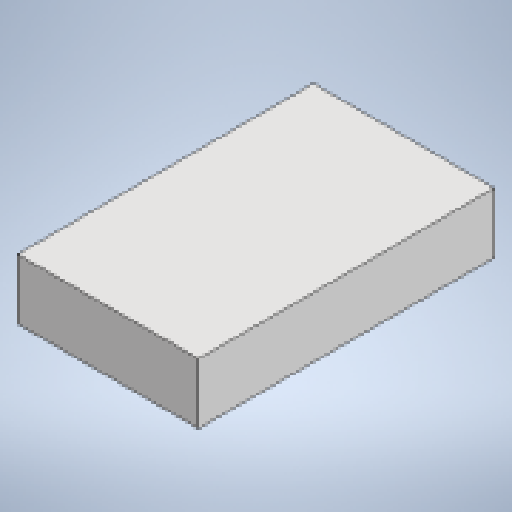
# Autodesk Inventor part: Temp - ESC
Saved by Autodesk Inventor 2023.2 (Build 272271000, 271)
## iProperties
Created: 2023-11-13
Part Number: Temp - ESC
Material: Generic
Document SubType Name: Modeling
Designer: Nathan Cai
Density: 1 g/cm^3
Appearance: Default
Author: Nathan Cai
Autodesk Inventor part; units mm, degrees
ref_plane "YZ Plane" through (0, 0, 0) normal (1, 0, 0) x (0, 1, 0)
ref_plane "XZ Plane" through (0, 0, 0) normal (0, 1, 0) x (-1, 0, 0)
ref_plane "XY Plane" through (0, 0, 0) normal (0, 0, 1) x (1, 0, 0)
sketch "Sketch1" plane through (0, 0, 0) normal (0, 1, 0) x (-1, 0, 0)
  line L0 (-15, 24.5) -> (15, 24.5)
  line L1 (15, 24.5) -> (15, -24.5)
  line L2 (15, -24.5) -> (-15, -24.5)
  line L3 (-15, -24.5) -> (-15, 24.5)
  line L4 (-15, 24.5) -> (15, -24.5) construction
  line L5 (15, 24.5) -> (-15, -24.5) construction
  point P0 (0, 0)
  dimension "d0" = 30
  dimension "d1" = 49
  constraints: 12 end point, 2 midpoint, 2 parallel, 1 horizontal, 1 perpendicular
  measures "d0" distance of L1.end L2.end
  measures "d1" distance of L0.end L1.end
extrude "Extrusion1" add sketch "Sketch1" along normal blind 10
body "Solid1"
